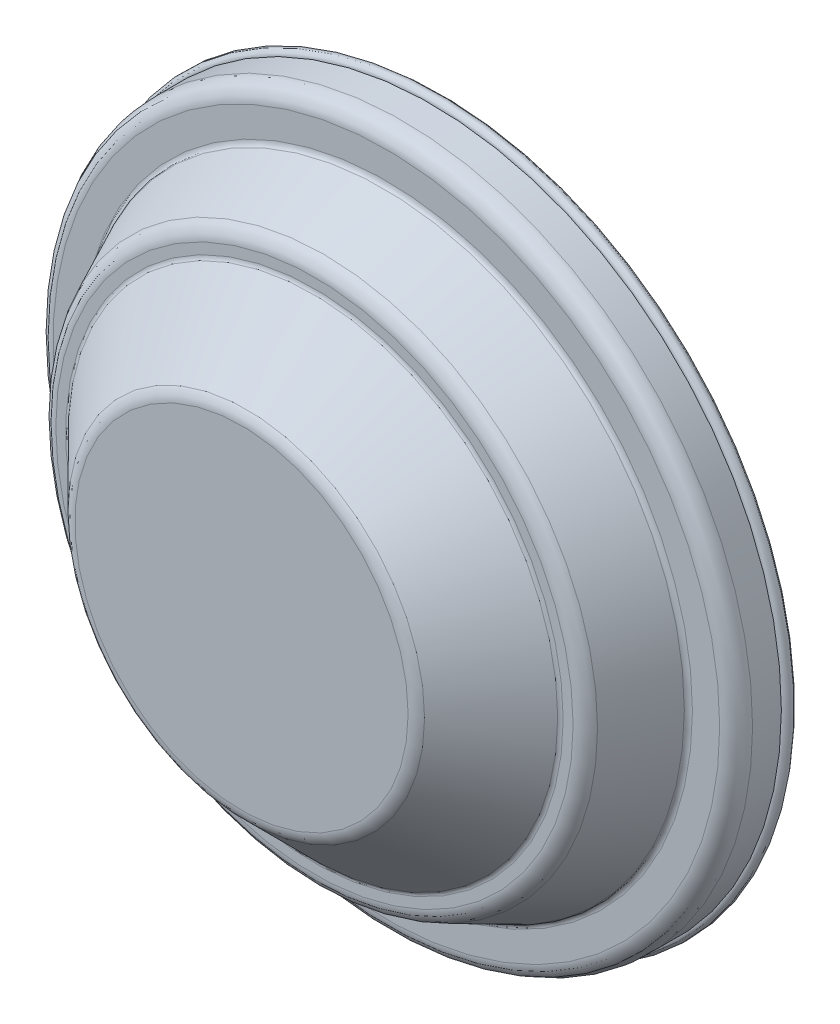
# Autodesk Inventor part: DisceepXL_Case
Saved by Autodesk Inventor 2014 (Build 180170000, 170)
## iProperties
Created: 2014-11-22
Part Number: DisceepXL_Case
Material: Polycarbonate, Smoke
Document SubType Name: Modeling
Designer: DV
Mass: 0.0548328 g
Surface Area: 7.26037 cm^2
Volume: 0.045694 cm^3
Density: 1.2 g/cm^3
Appearance: Polycarbonate - Smoked
Author: DV
Autodesk Inventor part; units mm, degrees
ref_plane "YZ Plane" through (0, 0, 0) normal (1, 0, 0) x (0, 1, 0)
ref_plane "XZ Plane" through (0, 0, 0) normal (0, 1, 0) x (-1, 0, 0)
ref_plane "XY Plane" through (0, 0, 0) normal (0, 0, 1) x (1, 0, 0)
sketch "Sketch1" plane through (0, 0, 0) normal (0, 0, 1) x (1, 0, 0)
  point P0 (0, 0)
sketch "Sketch2" plane through (0, 0, 0) normal (0, 1, 0) x (-1, 0, 0)
  line L0 (1.4612, -3.605) -> (-5.2946, -3.605) projected
  line L1 (6, 0) -> (-6, 0) projected
  line L2 (0, 1.6901) -> (-3.8591, 1.6901)
  line L3 (-4.0387, 1.6157) -> (-5.58, 0.0744)
  line L4 (-5.7596, 0) -> (-5.9897, 0)
  line L5 (-6.2199, -0.1467) -> (-6.8587, -1.5165)
  line L6 (-7.0889, -1.6632) -> (-7.7196, -1.6632)
  line L7 (-7.9736, -1.9172) -> (-7.9736, -2.7104)
  arc A0 (-3.8591, 1.6901) -> (-4.0387, 1.6157) centre (-3.8591, 1.4361) ccw
  arc A1 (-5.7596, 0) -> (-5.58, 0.0744) centre (-5.7596, 0.254) ccw
  arc A2 (-5.9897, 0) -> (-6.2199, -0.1467) centre (-5.9897, -0.254) ccw
  arc A3 (-7.0889, -1.6632) -> (-6.8587, -1.5165) centre (-7.0889, -1.4092) ccw
  arc A4 (-7.7196, -1.6632) -> (-7.9736, -1.9172) centre (-7.7196, -1.9172) ccw
  line L8 (0, 1.8171) -> (-3.8591, 1.8171)
  arc A5 (-3.8591, 1.8171) -> (-4.1285, 1.7055) centre (-3.8591, 1.4361) ccw
  line L9 (-4.1285, 1.7055) -> (-5.6698, 0.1642)
  arc A6 (-5.7596, 0.127) -> (-5.6698, 0.1642) centre (-5.7596, 0.254) ccw
  line L10 (-5.7596, 0.127) -> (-5.9897, 0.127)
  arc A7 (-5.9897, 0.127) -> (-6.335, -0.093) centre (-5.9897, -0.254) ccw
  line L11 (-6.335, -0.093) -> (-6.9738, -1.4629)
  arc A8 (-7.0889, -1.5362) -> (-6.9738, -1.4629) centre (-7.0889, -1.4092) ccw
  line L12 (-7.0889, -1.5362) -> (-7.7196, -1.5362)
  arc A9 (-7.7196, -1.5362) -> (-8.1006, -1.9172) centre (-7.7196, -1.9172) ccw
  line L13 (-8.1006, -1.9172) -> (-8.1006, -2.5834)
  line L14 (0, 1.6901) -> (0, 1.8171)
  arc A10 (-8.1006, -2.5834) -> (-7.9736, -2.7104) centre (-8.1006, -2.7104) ccw
  point P0 (0, 0)
  point P1 (-5.6544, 0)
  dimension "d0" = 45
  dimension "d1" = 115
  dimension "d2" = 0.254
  dimension "d3" = 0.127
  constraints: 26 end point, 22 point on circle, 11 centre point, 10 tangent, 5 parallel, 4 equal radius, 3 perpendicular, 3 point on line, 8 other
  measures "d0" angle of L1 L3
  measures "d1" angle of L6 L5
  measures "d2" radius of A0
  measures "d3" distance between parallel lines of L8 L2
revolve "Revolution1" add sketch "Sketch2" angle 360 about axis through (0, 0, 1.6901) along (0, 0, 1)
body "Solid1"
